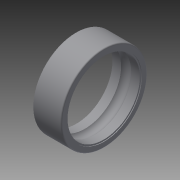
# Autodesk Inventor part: WBC6-12ZZ Outer ring
Saved by Autodesk Inventor 2014 SP2 (Build 180246200, 246)
## iProperties
Created: 2019-09-21
Part Number: WBC6-12ZZ Outer ring
Material: Generic
Catalog Web Link: www.cadenas.de
Description: Six types or-Metric system sizes
Vendor: NTN
Document SubType Name: Modeling
Designer: psadmin
Manufacturer: NTN
Mass: 0.120554 g
Surface Area: 3.48673 cm^2
Volume: 0.120554 cm^3
Density: 1 g/cm^3
Appearance: PSOLRGB-192-192-192
Category: PARTsolutions
Company: NTN
Title: WBC6-12ZZ Outer ring
Author: Cadenas PARTsolutions
Comments: Metric system sizes
PSOL_IDENT_0: {$CADENAS_DATA\23d-libs\ntn\ball_roller_bearings\miniature_extra_small_bb\metric_system_sizes\mss_or
PSOL_IDENT_1: .prj},189 {VTYP=3D},{NB=WBC6-12ZZ Outer ring},{LINA=WBC6-12ZZ Outer ring},{NN=Six types or},{DATE=29
PSOL_IDENT_2: .01.2019 23:03:33},{GEOMDATE=02.04.2007 00:00:00},{VERSION=},{LINEID=12850},{WBVAR=},{WBNUMERIC=}  {
PSOL_IDENT_3: NB=WBC6-12ZZ Outer ring},{LINA=WBC6-12ZZ Outer ring},{KT=DUMMY},{IDNR=},{SD=6.0},{D=12},{B=3.0},{R=0
PSOL_IDENT_4: .15},{ORDER=WBC6-12ZZ},{CR=830},{COR=365},{CRF=85},{CORF=37},{LSG=40 000},{LSO=47 000},{MASS=1.30},{
PSOL_IDENT_5: D1=13.2},{D2=13.6},{C1=0.6},{C2=0.8},{ORDER1=BC6-12},{WSS=WBC6-12ZZ},{WDS=ZZ},{UTWF=FLBC6-12},{FORSS=
PSOL_IDENT_6: FLAWBC6-12Z},{FORDS=ZZ},{DA1=7,2},{DA2=7,9},{DA=10,8},{RAS=0,15},{MASS1=1.40},{B1=4.0},{VERS=3},{X=3
PSOL_IDENT_7: },{N=9},{O=28.26},{RB=0.888}
NN: Six types or
NT: Metric system sizes
NB: WBC6-12ZZ Outer ring
NBSYN: $ORDER. Outer ring
LINA: WBC6-12ZZ Outer ring
SD: 6
D: 12
B: 3
R: 0.15
CR: 830
COR: 365
CRF: 85
CORF: 37
LSG: 40 000
LSO: 47 000
MASS: 1.3
D1: 13.2
D2: 13.6
C1: 0.6
C2: 0.8
ORDER1: BC6-12
WSS: WBC6-12ZZ
WDS: ZZ
UTWF: FLBC6-12
FORSS: FLAWBC6-12Z
FORDS: ZZ
DA1: 7,2
DA2: 7,9
DA: 10,8
RAS: 0,15
MASS1: 1.4
B1: 4
VERS: 3
SUPPLIER: NTN
ARTICLENO: WBC6-12ZZ Outer ring
BOMINFO: WBC6-12ZZ Outer ring
CREATOR: CADENAS GmbH
Autodesk Inventor part; units mm, degrees
sketch "Sketch_3" plane through (0, 0, 0) normal (0, 0, 1) x (1, 0, 0)
  line L0 (4, 0) -> (0, 0)
  line L1 (0, 5.232) -> (0.09, 5.232)
  line L2 (0.09, 5.232) -> (0.09, 5.04)
  line L3 (0.09, 5.04) -> (1.2951, 5.04)
  arc A0 (2.7049, 5.04) -> (1.2951, 5.04) centre (2, 4.5) ccw
  line L4 (2.7049, 5.04) -> (3.91, 5.04)
  line L5 (3.91, 5.04) -> (3.91, 5.232)
  line L6 (3.91, 5.232) -> (4, 5.232)
  line L7 (4, 5.232) -> (4, 5.85)
  arc A1 (4, 5.85) -> (3.85, 6) centre (3.85, 5.85) ccw
  line L8 (3.85, 6) -> (0.15, 6)
  arc A2 (0.15, 6) -> (0, 5.85) centre (0.15, 5.85) ccw
  line L9 (0, 5.85) -> (0, 5.232)
  constraints: 20 end point, 6 point on circle, 3 centre point
revolve "Revolution1" add sketch "Sketch_3" angle 360 about axis through (4, 0, 0) along (1, 0, 0)
ref_plane "mss_or_XY" through (0, 0, 0) normal (1, 0, 0) x (0, 0, -1)
ref_plane "mss_or_YZ" through (0, 0, 0) normal (0, 0, -1) x (0, 1, 0)
ref_plane "mss_or_ZX" through (0, 0, 0) normal (0, 1, 0) x (1, 0, 0)
ref_plane "mss_or11_XY" through (4, 0, 0) normal (1, 0, 0) x (0, 0, -1)
ref_plane "mss_or11_YZ" through (4, 0, 0) normal (0, 0, -1) x (0, 1, 0)
ref_plane "mss_or11_ZX" through (4, 0, 0) normal (0, 1, 0) x (1, 0, 0)
ref_plane "mss_or2_1_XY" through (1.5, 4.5, 0) normal (1, 0, 0) x (0, 0, -1)
ref_plane "mss_or2_1_YZ" through (1.5, 4.5, 0) normal (0, 0, -1) x (0, 1, 0)
ref_plane "mss_or2_1_ZX" through (1.5, 4.5, 0) normal (0, 1, 0) x (1, 0, 0)
ref_plane "mss_or2_2_XY" through (1.5, 3.4472, 2.8925) normal (1, 0, 0) x (0, 0, -1)
ref_plane "mss_or2_2_YZ" through (1.5, 3.4472, 2.8925) normal (0, 0, -1) x (0, 1, 0)
ref_plane "mss_or2_2_ZX" through (1.5, 3.4472, 2.8925) normal (0, 1, 0) x (1, 0, 0)
ref_plane "mss_or2_3_XY" through (1.5, 0.7814, 4.4316) normal (1, 0, 0) x (0, 0, -1)
ref_plane "mss_or2_3_YZ" through (1.5, 0.7814, 4.4316) normal (0, 0, -1) x (0, 1, 0)
ref_plane "mss_or2_3_ZX" through (1.5, 0.7814, 4.4316) normal (0, 1, 0) x (1, 0, 0)
ref_plane "mss_or2_4_XY" through (1.5, -2.25, 3.8971) normal (1, 0, 0) x (0, 0, -1)
ref_plane "mss_or2_4_YZ" through (1.5, -2.25, 3.8971) normal (0, 0, -1) x (0, 1, 0)
ref_plane "mss_or2_4_ZX" through (1.5, -2.25, 3.8971) normal (0, 1, 0) x (1, 0, 0)
ref_plane "mss_or2_5_XY" through (1.5, -4.2286, 1.5391) normal (1, 0, 0) x (0, 0, -1)
ref_plane "mss_or2_5_YZ" through (1.5, -4.2286, 1.5391) normal (0, 0, -1) x (0, 1, 0)
ref_plane "mss_or2_5_ZX" through (1.5, -4.2286, 1.5391) normal (0, 1, 0) x (1, 0, 0)
ref_plane "mss_or2_6_XY" through (1.5, -4.2286, -1.5391) normal (1, 0, 0) x (0, 0, -1)
ref_plane "mss_or2_6_YZ" through (1.5, -4.2286, -1.5391) normal (0, 0, -1) x (0, 1, 0)
ref_plane "mss_or2_6_ZX" through (1.5, -4.2286, -1.5391) normal (0, 1, 0) x (1, 0, 0)
ref_plane "mss_or2_7_XY" through (1.5, -2.25, -3.8971) normal (1, 0, 0) x (0, 0, -1)
ref_plane "mss_or2_7_YZ" through (1.5, -2.25, -3.8971) normal (0, 0, -1) x (0, 1, 0)
ref_plane "mss_or2_7_ZX" through (1.5, -2.25, -3.8971) normal (0, 1, 0) x (1, 0, 0)
ref_plane "mss_or2_8_XY" through (1.5, 0.7814, -4.4316) normal (1, 0, 0) x (0, 0, -1)
ref_plane "mss_or2_8_YZ" through (1.5, 0.7814, -4.4316) normal (0, 0, -1) x (0, 1, 0)
ref_plane "mss_or2_8_ZX" through (1.5, 0.7814, -4.4316) normal (0, 1, 0) x (1, 0, 0)
ref_plane "mss_or2_9_XY" through (1.5, 3.4472, -2.8925) normal (1, 0, 0) x (0, 0, -1)
ref_plane "mss_or2_9_YZ" through (1.5, 3.4472, -2.8925) normal (0, 0, -1) x (0, 1, 0)
ref_plane "mss_or2_9_ZX" through (1.5, 3.4472, -2.8925) normal (0, 1, 0) x (1, 0, 0)
ref_plane "mss_or21_1_XY" through (2, 4.5, 0) normal (1, 0, 0) x (0, 0, -1)
ref_plane "mss_or21_1_YZ" through (2, 4.5, 0) normal (0, 0, -1) x (0, 1, 0)
ref_plane "mss_or21_1_ZX" through (2, 4.5, 0) normal (0, 1, 0) x (1, 0, 0)
ref_plane "mss_or21_2_XY" through (2, 3.4472, 2.8925) normal (1, 0, 0) x (0, 0, -1)
ref_plane "mss_or21_2_YZ" through (2, 3.4472, 2.8925) normal (0, 0, -1) x (0, 1, 0)
ref_plane "mss_or21_2_ZX" through (2, 3.4472, 2.8925) normal (0, 1, 0) x (1, 0, 0)
ref_plane "mss_or21_3_XY" through (2, 0.7814, 4.4316) normal (1, 0, 0) x (0, 0, -1)
ref_plane "mss_or21_3_YZ" through (2, 0.7814, 4.4316) normal (0, 0, -1) x (0, 1, 0)
ref_plane "mss_or21_3_ZX" through (2, 0.7814, 4.4316) normal (0, 1, 0) x (1, 0, 0)
ref_plane "mss_or21_4_XY" through (2, -2.25, 3.8971) normal (1, 0, 0) x (0, 0, -1)
ref_plane "mss_or21_4_YZ" through (2, -2.25, 3.8971) normal (0, 0, -1) x (0, 1, 0)
ref_plane "mss_or21_4_ZX" through (2, -2.25, 3.8971) normal (0, 1, 0) x (1, 0, 0)
ref_plane "mss_or21_5_XY" through (2, -4.2286, 1.5391) normal (1, 0, 0) x (0, 0, -1)
ref_plane "mss_or21_5_YZ" through (2, -4.2286, 1.5391) normal (0, 0, -1) x (0, 1, 0)
ref_plane "mss_or21_5_ZX" through (2, -4.2286, 1.5391) normal (0, 1, 0) x (1, 0, 0)
ref_plane "mss_or21_6_XY" through (2, -4.2286, -1.5391) normal (1, 0, 0) x (0, 0, -1)
ref_plane "mss_or21_6_YZ" through (2, -4.2286, -1.5391) normal (0, 0, -1) x (0, 1, 0)
ref_plane "mss_or21_6_ZX" through (2, -4.2286, -1.5391) normal (0, 1, 0) x (1, 0, 0)
ref_plane "mss_or21_7_XY" through (2, -2.25, -3.8971) normal (1, 0, 0) x (0, 0, -1)
ref_plane "mss_or21_7_YZ" through (2, -2.25, -3.8971) normal (0, 0, -1) x (0, 1, 0)
ref_plane "mss_or21_7_ZX" through (2, -2.25, -3.8971) normal (0, 1, 0) x (1, 0, 0)
ref_plane "mss_or21_8_XY" through (2, 0.7814, -4.4316) normal (1, 0, 0) x (0, 0, -1)
ref_plane "mss_or21_8_YZ" through (2, 0.7814, -4.4316) normal (0, 0, -1) x (0, 1, 0)
ref_plane "mss_or21_8_ZX" through (2, 0.7814, -4.4316) normal (0, 1, 0) x (1, 0, 0)
ref_plane "mss_or21_9_XY" through (2, 3.4472, -2.8925) normal (1, 0, 0) x (0, 0, -1)
ref_plane "mss_or21_9_YZ" through (2, 3.4472, -2.8925) normal (0, 0, -1) x (0, 1, 0)
ref_plane "mss_or21_9_ZX" through (2, 3.4472, -2.8925) normal (0, 1, 0) x (1, 0, 0)
body "Solid1"
